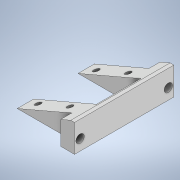
# Autodesk Inventor part: Camera Angle
Saved by Autodesk Inventor 2022 (Build 260153000, 153)
## iProperties
Created: 2023-03-09
Part Number: Camera Angle
Material: Generic
Document SubType Name: Modeling
Designer: zarek
Density: 1 g/cm^3
Appearance: Default
Author: zarek
Autodesk Inventor part; units mm, degrees
ref_plane "YZ Plane" through (0, 0, 0) normal (1, 0, 0) x (0, 1, 0)
ref_plane "XZ Plane" through (0, 0, 0) normal (0, 1, 0) x (-1, 0, 0)
sketch "Sketch2" plane through (0, 0, 0) normal (0, 1, 0) x (-1, 0, 0)
  line L0 (0, 0) -> (23.273, 0)
  line L1 (23.273, 0) -> (23.273, -37.9053)
  line L2 (23.273, -37.9053) -> (0, -37.9053)
  line L3 (0, -37.9053) -> (0, 0)
  line L4 (26.75, 0) -> (-5, 0)
  line L5 (-5, 0) -> (-5, -37.9053)
  line L6 (-5, -37.9053) -> (26.75, -37.9053)
  line L7 (26.75, -37.9053) -> (26.75, 0)
  point P0 (0, -37.9053)
  dimension "d21" = 37.9053
  dimension "d22" = 23.273
  dimension "d36" = 5
  dimension "d37" = 31.75
  constraints: 16 end point, 4 parallel, 2 horizontal, 2 perpendicular
  measures "d21" distance between parallel lines of L2 L0
  measures "d22" distance of L1.end L2.end
  measures "d36" distance between parallel lines of L5 L3
  measures "d37" distance between parallel lines of L5 L7
extrude "Extrusion1" add sketch "Sketch2" along normal blind 10
sketch "Sketch6" plane through (-26.75, 0, 0) normal (0, 0, 1) x (1, 0, 0)
  line L0 (31.75, 0) -> (31.75, 10) projected
  line L1 (31.75, 0) -> (31.75, 10)
  line L2 (31.75, 0) -> (0, 0) projected
  line L3 (30.3918, 0) -> (30.3918, 10)
  line L4 (31.75, 10) -> (0, 10) projected
  line L5 (30.3918, 10) -> (55.3918, 10) construction
  line L6 (0, 0) -> (0, 10) projected
  line L7 (0, 0) -> (0, 0.5)
  line L8 (30.3918, 10) -> (7.0432, 0)
  point P0 (26.75, 0)
  dimension "d38" = 1.3582
  dimension "d41" = 0.5
  dimension "d96" = 25.4
  dimension "d97" = 66.815
  constraints: 10 end point, 4 point on line, 2 vertical, 1 horizontal
  measures "d38" distance between parallel lines of L0 L3
  measures "d41" distance of L2.end L7.end
  measures "d96" distance of L3.end L8.end
  measures "d97" angle of L3 L8
extrude "Extrusion2" cut sketch "Sketch6" against normal up to surface (37.9053 mm away) contours L8 L2 L6 L4
sketch "Sketch8" plane through (0, 0, 0) normal (0, -1, 0) x (1, 0, 0)
  line L0 (-26.75, -37.9053) -> (-26.75, 0) projected
  line L1 (-26.75, -10.922) -> (3, -10.922)
  line L2 (3, -10.922) -> (3, -26.9833)
  line L3 (3, -26.9833) -> (-26.75, -26.9833)
  line L4 (-26.75, -26.9833) -> (-26.75, -10.922)
  line L5 (-26.75, 0) -> (5, 0) projected
  line L6 (5, -37.9053) -> (-26.75, -37.9053) projected
  line L7 (5, 0) -> (5, -37.9053) projected
  point P0 (0, 0)
  point P1 (-26.75, -26.9833)
  dimension "d44" = 10.922
  dimension "d45" = 10.922
  dimension "d46" = 2
  constraints: 8 end point, 2 parallel, 1 horizontal, 1 perpendicular, 1 point on line
  measures "d44" distance between parallel lines of L1 L5
  measures "d45" distance between parallel lines of L6 L3
  measures "d46" distance between parallel lines of L7 L2
extrude "Extrusion3" cut sketch "Sketch8" against normal blind 25.4 contours L0 L1 L2 L3
ref_plane "Work Plane1" through (4.3209, 10, 0) normal (0, 1, 0) x (1, 0, 0)
sketch "Sketch12" plane through (0, 0, 0) normal (0, -1, 0) x (1, 0, 0)
  line L0 (3.6418, 0) -> (-26.75, 0) projected
  line L1 (-26.75, 0) -> (0, 0)
  line L2 (0, 0) -> (0, -5)
  line L3 (0, -5) -> (-26.75, -5)
  line L4 (-26.75, -5) -> (-26.75, 0)
  line L5 (-26.75, -37.9053) -> (0, -37.9053)
  line L6 (0, -37.9053) -> (0, -32.9053)
  line L7 (0, -32.9053) -> (-26.75, -32.9053)
  line L8 (-26.75, -32.9053) -> (-26.75, -37.9053)
  line L9 (5, 0) -> (0, 0)
  line L10 (0, 0) -> (0, -1)
  line L11 (0, -1) -> (5, -1)
  line L12 (5, -1) -> (5, 0)
  line L13 (5, 0) -> (5, -37.9053) projected
  line L14 (5, -37.9053) -> (0, -37.9053)
  line L15 (0, -37.9053) -> (0, -36.9053)
  line L16 (0, -36.9053) -> (5, -36.9053)
  line L17 (5, -36.9053) -> (5, -37.9053)
  line L18 (5, -37.9053) -> (-26.75, -37.9053) projected
  point P0 (0, -37.9053)
  dimension "d69" = 5
  dimension "d70" = 5
  dimension "d73" = 1
  dimension "d74" = 1
  dimension "d75" = 0
  constraints: 32 end point, 8 parallel, 4 horizontal, 4 perpendicular, 4 point on line
  measures "d69" distance between parallel lines of L3 L0
  measures "d70" distance between parallel lines of L5 L7
  measures "d73" distance of L10.end L9.end
  measures "d74" distance of L14.end L15.end
  measures "d75" distance between parallel lines of L5 L18
extrude "Extrusion6" cut sketch "Sketch12" along normal through all both and the other way through all
sketch "Sketch13" plane through (0, 0, -36.9053) normal (-1, 0, 0) x (0, 0, 1)
  circle A0 centre (2, 3.9204) radius 1.5
  circle A1 centre (33.9053, 3.9204) radius 1.5
  line L0 (35.9053, 0) -> (31.9053, 0) projected
  line L1 (31.9053, 7.8408) -> (35.9053, 7.8408) projected
  line L2 (35.9053, 8.4402) -> (35.9053, 0) projected
  line L3 (31.9053, 2) -> (31.9053, 7.8408) projected
  line L4 (0, 0) -> (0, 8.4402) projected
  line L5 (0, 7.8408) -> (4, 7.8408) projected
  line L6 (4, 0) -> (0, 0) projected
  point P0 (36.9053, 0)
  point P1 (35.9053, 8.636)
  point P2 (0, 8.636)
  dimension "d80" = 3
  dimension "d81" = 3
  dimension "d82" = 7.8408
  dimension "d83" = 3.9204
  dimension "d84" = 4
  dimension "d85" = 2
  dimension "d86" = 2
  dimension "d87" = 3.9204
  dimension "d88" = 31.9053
  dimension "d148" = 3.9204
  constraints: 2 centre point
  measures "d80" diameter of A0
  measures "d81" diameter of A1
  measures "d82" distance between parallel lines of L0 L1
  measures "d83" distance from line of A1.centre L1
  measures "d84" distance between parallel lines of L2 L3
  measures "d85" distance from line of L2 A1.centre
  measures "d86" distance from line of L4 A0.centre
  measures "d87" distance from line of A0.centre L5
  measures "d88" distance of A1.centre A0.centre
  measures "d148" distance from line of L6 A0.centre
extrude "Extrusion7" cut sketch "Sketch13" against normal blind 25.4
sketch "Sketch15" plane through (3, 9.7251, -10.922) normal (-0.3937008, 0.9192386, 0) x (0.9192386, 0.3937008, 0)
  circle A0 centre (-20.2819, -2.4315) radius 1.1146
  circle A1 centre (-7.7426, 18.5871) radius 1.229
  line L0 (-20.2819, -2.4315) -> (-20.2819, 18.5871)
  line L1 (-20.2819, 18.5871) -> (-7.7426, 18.5871)
  line L2 (-7.7426, 18.5871) -> (-7.7426, -2.4315)
  line L3 (-7.7426, -2.4315) -> (-20.2819, -2.4315)
  line L4 (-12.8147, 2.62) -> (-12.8147, 13.4413)
  line L5 (-12.8147, 13.4413) -> (-2.3681, 13.4413)
  line L6 (-2.3681, 13.4413) -> (-2.3681, 2.62)
  line L7 (-2.3681, 2.62) -> (-12.8147, 2.62)
  line L8 (-22.0533, -4.4694) -> (-22.0533, 20.5306)
  line L9 (-22.0533, 20.5306) -> (1.9467, 20.5306)
  line L10 (1.9467, 20.5306) -> (1.9467, -4.4694)
  line L11 (1.9467, -4.4694) -> (-22.0533, -4.4694)
  line L12 (-3.2636, 21.9833) -> (-24.7018, 21.9833) projected
  line L13 (-24.7018, -5.922) -> (-3.2636, -5.922) projected
  circle A2 centre (-20.2819, 18.5871) radius 1.1245
  line L14 (0, 16.0613) -> (0, 0) projected
  line L15 (1.9467, -9.922) -> (1.9467, 25.9833) projected
  circle A3 centre (-7.7426, -2.4315) radius 1.1245
  point P0 (-6.5865, -10.922)
  dimension "d107" = 21.0186
  dimension "d108" = 12.5392
  dimension "d110" = 25
  dimension "d111" = 24
  dimension "d112" = 4.3148
  dimension "d113" = 9.2386
  dimension "d114" = 7.0893
  dimension "d115" = 7.0893
  dimension "d117" = 1.9436
  dimension "d118" = 2.0378
  dimension "d119" = 1.7714
  dimension "d120" = 9.6893
  dimension "d122" = 1.4526
  dimension "d123" = 1.4526
  dimension "d124" = 2.249
  dimension "d133" = 0
  dimension "d134" = 2.249
  constraints: 24 end point, 6 parallel, 4 centre point, 3 perpendicular, 2 coincident
  measures "d107" distance of L0.start L0.end
  measures "d108" distance of L0.end L1.end
  measures "d110" distance between parallel lines of L9 L11
  measures "d111" distance between parallel lines of L10 L8
  measures "d112" distance between parallel lines of L10 L6
  measures "d113" distance between parallel lines of L4 L8
  measures "d114" distance between parallel lines of L11 L7
  measures "d115" distance between parallel lines of L9 L5
  measures "d117" distance between parallel lines of L1 L9
  measures "d118" distance between parallel lines of L11 L3
  measures "d119" distance between parallel lines of L8 L0
  measures "d120" distance between parallel lines of L10 L2
  measures "d122" distance between parallel lines of L9 L12
  measures "d123" distance between parallel lines of L13 L11
  measures "d124" diameter of A2
  measures "d133" distance between parallel lines of L15 L10
  measures "d134" diameter of A3
hole "Hole3" at (-15.6439, 1.7401, -8.4905) at (-4.1173, 6.6768, -8.4905) at (-4.1173, 6.6768, -29.5091) at (-15.6439, 1.7401, -29.5091) direction (0.3937008, -0.9192386, 0) diameter 2.1211 depth 7.1 tip angle 118 countersink diameter 2.125 countersink angle 90 thread size "M2.5x0.35" class "6H" standard "ANSI Metric M Profile"
chamfer "Chamfer3" distance 2 distance2 2 1 edges at (3, 0, -18.9526) measured on face at (4.3333, 0, -21.6295)
equation "\"d83\" = 0.5 * d82"
equation "\"d85\" = 0.5 * d84"
equation "\"d86\" = d85"
equation "\"d87\" = d83"
equation "\"d115\" = d114"
equation "\"d122\" = d123"
body "Solid1"
